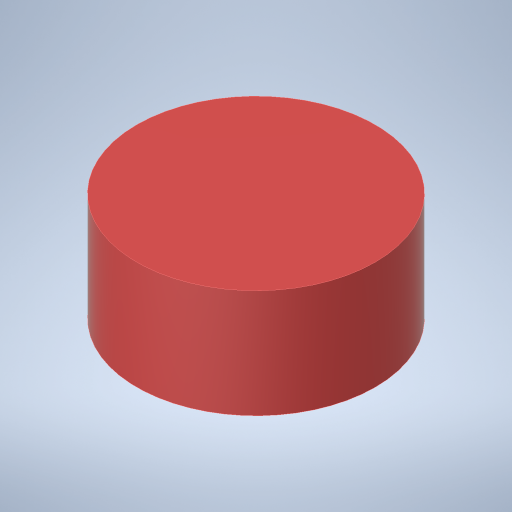
# Autodesk Inventor part: CLIMBER LATCH SPACER
Saved by Autodesk Inventor 2023.4 (Build 274418000, 418)
## iProperties
Created: 2025-03-24
Part Number: CLIMBER LATCH SPACER
Material: ABS Plastic
Document SubType Name: Modeling
Designer: jmcintyr
Density: 1.06 g/cm^3
Appearance: Smooth - Red
Author: jmcintyr
Autodesk Inventor part; units mm, degrees
ref_plane "YZ Plane" through (0, 0, 0) normal (1, 0, 0) x (0, 1, 0)
ref_plane "XZ Plane" through (0, 0, 0) normal (0, 1, 0) x (-1, 0, 0)
ref_plane "XY Plane" through (0, 0, 0) normal (0, 0, 1) x (1, 0, 0)
sketch "Sketch1" plane through (0, 0, 0) normal (0, 1, 0) x (-1, 0, 0)
  circle A0 centre (0, 0) radius 8.7312
  dimension "d0" = 17.4625
  constraints: 1 centre point, 1 coincident
  measures "d0" diameter of A0
extrude "Extrusion1" add sketch "Sketch1" along normal mid plane 7.9375
body "Solid1"
